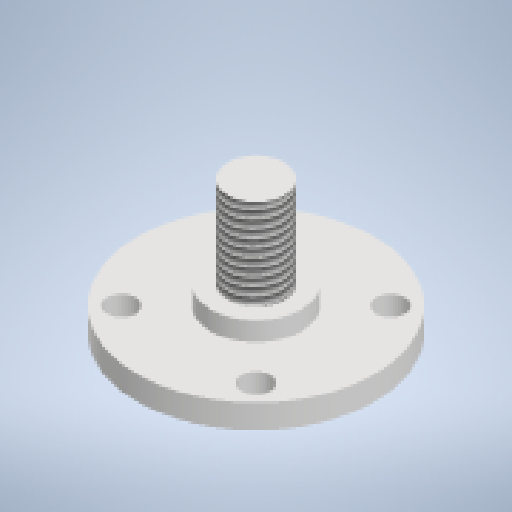
# Autodesk Inventor part: PortaMandril
Saved by Autodesk Inventor 2023.1 (Build 271208000, 208)
## iProperties
Created: 2022-08-26
Part Number: PortaMandril
Material: Generic
Document SubType Name: Modeling
Designer: danie_p
Density: 1 g/cm^3
Appearance: Default
Author: danie_p
Autodesk Inventor part; units mm, degrees
ref_plane "YZ Plane" through (0, 0, 0) normal (1, 0, 0) x (0, 1, 0)
ref_plane "XZ Plane" through (0, 0, 0) normal (0, 1, 0) x (-1, 0, 0)
ref_plane "XY Plane" through (0, 0, 0) normal (0, 0, 1) x (1, 0, 0)
sketch "Sketch1" plane through (0, 0, 0) normal (0, 1, 0) x (-1, 0, 0)
  circle A0 centre (0, 0) radius 25
  dimension "d0" = 50
  constraints: 1 centre point, 1 coincident
  measures "d0" diameter of A0
extrude "Extrusion1" add sketch "Sketch1" along normal blind 5
sketch "Sketch2" plane through (0, 5, 0) normal (0, 1, 0) x (1, 0, 0)
  line L0 (0, 0) -> (-14.1421, -14.1421) construction
  line L1 (0, 0) -> (20, 0) construction
  point P0 (14.1421, -14.1421)
  point P1 (14.1421, 14.1421)
  point P2 (-14.1421, 14.1421)
  dimension "d3" = 20
  dimension "d4" = 135
  dimension "d7" = 360
  constraints: 4 end point, 1 coincident, 1 equal length, 1 horizontal, 5 other
  measures "d3" distance of L0.start L0.end
  measures "d4" angle of L0 L1
hole "Hole1" at (-14.1421, 5, 14.1421) at (14.1421, 5, 14.1421) at (14.1421, 5, -14.1421) at (-14.1421, 5, -14.1421) direction (0, -1, 0) diameter 6 end through all
sketch "Sketch3" plane through (0, 5, 0) normal (0, 1, 0) x (1, 0, 0)
  circle A0 centre (0, 0) radius 9.5
  dimension "d16" = 19
  constraints: 1 centre point, 1 coincident
  measures "d16" diameter of A0
extrude "Extrusion2" add sketch "Sketch3" along normal blind 4
sketch "Sketch4" plane through (0, 9, 0) normal (0, 1, 0) x (1, 0, 0)
  circle A0 centre (0, 0) radius 6
  dimension "d19" = 12
  constraints: 1 centre point, 1 coincident
  measures "d19" diameter of A0
extrude "Extrusion3" add sketch "Sketch4" along normal blind 19
thread "Thread1" size "M12x1.75" class "6g" standard "ANSI Metric M Profile" full length
body "Solid1"
